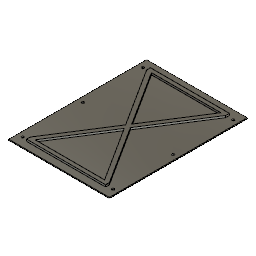
smmb_back (Autodesk Fusion 360 design; units mm, degrees)
Autodesk Fusion 360 part; units mm, degrees
sketch "Sketch1" plane through (0, 0, 0) normal (0, 0, 1) x (1, 0, 0)
  line L0 (0, 0) -> (134, 0)
  line L1 (134, 0) -> (134, 183.541)
  line L2 (134, 183.541) -> (0, 183.541)
  line L3 (0, 183.541) -> (0, 0)
  circle A0 centre (7, 171.541) radius 1.55
  circle A1 centre (7, 12) radius 1.55
  circle A2 centre (7, 91.771) radius 1.55
  line L4 (67, 0) -> (67, 183.541) construction
  circle A3 centre (127, 12) radius 1.55
  circle A4 centre (127, 91.771) radius 1.55
  circle A5 centre (127, 171.541) radius 1.55
  line L5 (119.5, 174.041) -> (14.5, 174.041)
  line L6 (14.5, 174.041) -> (14.5, 169.041)
  line L7 (14.5, 169.041) -> (119.5, 169.041)
  line L8 (119.5, 169.041) -> (119.5, 174.041)
  line L9 (119.5, 174.041) -> (14.5, 169.041) construction
  line L10 (14.5, 174.041) -> (119.5, 169.041) construction
  line L11 (119.5, 9.5) -> (14.5, 9.5)
  line L12 (14.5, 9.5) -> (14.5, 14.5)
  line L13 (14.5, 14.5) -> (119.5, 14.5)
  line L14 (119.5, 14.5) -> (119.5, 9.5)
  line L15 (119.5, 9.5) -> (14.5, 14.5) construction
  line L16 (14.5, 9.5) -> (119.5, 14.5) construction
  line L17 (14.5, 9.5) -> (119.5, 174.041)
  line L18 (14.5, 14.5) -> (116.3093, 174.041)
  line L19 (119.5, 169.041) -> (17.6907, 9.5)
  line L20 (14.5, 174.041) -> (119.5, 9.5)
  line L21 (119.5, 14.5) -> (17.6907, 174.041)
  line L22 (14.5, 169.041) -> (116.3093, 9.5)
  point P0 (67, 171.541)
  point P1 (67, 12)
  dimension "d1" = 183.541
  dimension "d2" = 134
  dimension "d3" = 3.1
  dimension "d4" = 7
  dimension "d5" = 12
  dimension "d6" = 3.1
  dimension "d7" = 7
  dimension "d8" = 12
  dimension "d9" = 3.1
  dimension "d10" = 7
  dimension "d11" = 91.77
  dimension "d12" = 105
  dimension "d13" = 5
  dimension "d14" = 105
  dimension "d15" = 5
  constraint horizontal L0
  constraint vertical L1
  constraint horizontal L2
  constraint vertical L3
  constraint coincident L0.start L3.end
  constraint midpoint L0 L4.start
  constraint perpendicular L0 L4
  constraint midpoint L2 L4.end
  constraint symmetric A0 L4 A5
  constraint symmetric A1 L4 A3
  constraint symmetric A2 L4 A4
  constraint perpendicular L5 L6
  constraint parallel L5 L7
  constraint parallel L6 L8
  constraint horizontal L5
  constraint coincident L9 P0
  constraint coincident L10 P0
  constraint coincident L4 P0
  constraint perpendicular L11 L12
  constraint parallel L11 L13
  constraint parallel L12 L14
  constraint horizontal L11
  constraint coincident L15 P1
  constraint coincident L16 P1
  constraint coincident L4 P1
  constraint parallel L17 L18
  constraint coincident L5 L18.end
  constraint parallel L17 L19
  constraint coincident L11 L19.end
  constraint coincident L5 L21.end
  constraint parallel L20 L21
  constraint coincident L11 L22.end
  constraint parallel L21 L22
  measures "d1" distance of L0.start L2.end
  measures "d2" distance of L0.start L0.end
  measures "d3" diameter of A0
  measures "d4" distance of L3 A0.centre
  measures "d5" distance of L2 A0.centre
  measures "d6" diameter of A1
  measures "d7" distance of L3 A1.centre
  measures "d8" distance of L0 A1.centre
  measures "d9" diameter of A2
  measures "d10" distance of L3 A2.centre
  measures "d11" distance of L2 A2.centre
  measures "d12" distance of L6.end L7.end
  measures "d13" distance of L5.end L6.end
  measures "d14" distance of L12.end L13.end
  measures "d15" distance of L11.end L12.end
extrude "Extrude1" add sketch "Sketch1" along normal blind 1.5 contours L0 L1 L2 L3 | L5 L7 L17 L18 | L7 L8 L17 | L5 L7 L18 L21 | L7 L17 L19 L21 | L7 L17 L18 L21 | L5 L7 L20 L21 | L7 L18 L21 | L13 L19 L20 L21 | L17 L19 L20 L21 | L17 L18 L20 L21 | L6 L7 L20 | L7 L18 L20 L21 | L13 L19 L20 L22 | L17 L19 L20 L22 | L13 L14 L20 | L17 L18 L20 L22 | L7 L18 L20 L22 | L13 L19 L22 | L13 L17 L19 L22 | L11 L13 L20 L22 | L13 L17 L18 L22 | L11 L13 L17 L19 | L11 L13 L19 L22 | L12 L13 L17
extrude "Extrude2" add sketch "Sketch1" along normal blind 4 contours L5 L7 L17 L18 | L7 L8 L17 | L5 L7 L18 L21 | L7 L17 L19 L21 | L7 L17 L18 L21 | L5 L7 L20 L21 | L13 L19 L20 L21 | L17 L19 L20 L21 | L17 L18 L20 L21 | L6 L7 L20 | L7 L18 L20 L21 | L13 L19 L20 L22 | L17 L19 L20 L22 | L13 L14 L20 | L17 L18 L20 L22 | L7 L18 L20 L22 | L13 L17 L19 L22 | L11 L13 L20 L22 | L13 L17 L18 L22 | L11 L13 L17 L19 | L11 L13 L19 L22 | L12 L13 L17
equation "d6 = d3"
equation "d7 = d4"
equation "d8 = d5"
equation "d9 = d3"
